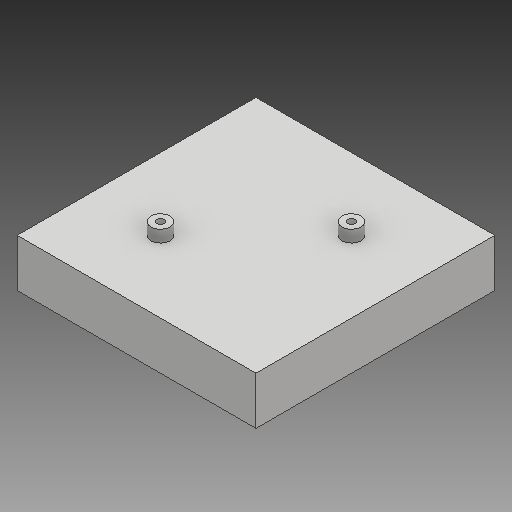
# Autodesk Inventor part: platine
Saved by Autodesk Inventor 2019 (Build 230136000, 136)
## iProperties
Created: 2018-07-23
Part Number: platine
Material: Generisch
Document SubType Name: Modeling
Designer: juliu
Density: 1 g/cm^3
Appearance: Vorgabe
Author: juliu
Autodesk Inventor part; units mm, degrees
ref_plane "YZ Plane" through (0, 0, 0) normal (1, 0, 0) x (0, 1, 0)
ref_plane "XZ Plane" through (0, 0, 0) normal (0, 1, 0) x (-1, 0, 0)
ref_plane "XY Plane" through (0, 0, 0) normal (0, 0, 1) x (1, 0, 0)
sketch "Skizze1" plane through (0, 0, 0) normal (0, 0, 1) x (1, 0, 0)
  line L0 (0, 0) -> (100, 0)
  line L1 (100, 0) -> (100, 100)
  line L2 (100, 100) -> (0, 100)
  line L3 (0, 100) -> (0, 0)
  dimension "d0" = 100
  dimension "d1" = 100
  constraints: 8 end point, 2 parallel, 1 horizontal, 1 perpendicular
  measures "d0" distance of L1.end L2.end
  measures "d1" distance of L0.end L1.end
extrude "Extrusion1" add sketch "Skizze1" along normal blind 20
sketch "Skizze2" plane through (0, 0, 20) normal (0, 0, 1) x (1, 0, 0)
  line L0 (0, 0) -> (100, 0) projected
  line L1 (0, 100) -> (0, 0) projected
  line L2 (100, 100) -> (0, 100) projected
  line L3 (100, 0) -> (100, 100) projected
  point P0 (30, 30)
  point P1 (70, 70)
  dimension "d4" = 30
  dimension "d5" = 30
  dimension "d6" = 30
  dimension "d7" = 30
  measures "d4" distance from line of L0 point (30, 30)
  measures "d5" distance from line of L1 point (30, 30)
  measures "d6" distance from line of L2 point (70, 70)
  measures "d7" distance from line of L3 point (70, 70)
hole "Bohrung1" at (30, 30, 20) at (70, 70, 20) direction (0, 0, -1) diameter 3 end through all
sketch "Skizze3" plane through (0, 0, 20) normal (0, 0, 1) x (1, 0, 0)
  circle A0 centre (30, 30) radius 1.5
  circle A1 centre (30, 30) radius 4
  circle A2 centre (30, 30) radius 1.5 projected
  point P0 (0, 0)
  dimension "d15" = 3
  dimension "d16" = 8
  constraints: 2 centre point, 1 coincident, 1 concentric
  measures "d15" diameter of A0
  measures "d16" diameter of A1
extrude "Extrusion2" add sketch "Skizze3" along normal blind 5
sketch "Skizze4" plane through (0, 0, 20) normal (0, 0, 1) x (1, 0, 0)
  circle A0 centre (70, 70) radius 4
  circle A1 centre (70, 70) radius 1.5
  circle A2 centre (70, 70) radius 1.5 projected
  circle A3 centre (70, 70) radius 1.5 projected
  point P0 (0, 0)
  dimension "d19" = 3
  dimension "d20" = 8
  constraints: 2 centre point, 1 coincident, 1 concentric
  measures "d19" diameter of A1
  measures "d20" diameter of A0
extrude "Extrusion3" add sketch "Skizze4" along normal blind 5
